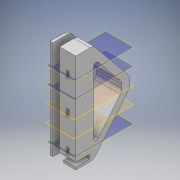
# Autodesk Inventor part: bumper_backright
Saved by Autodesk Inventor 2018 (Build 220112000, 112)
## iProperties
Created: 2019-04-08
Part Number: bumper_backright
Material: Generic
Document SubType Name: Modeling
Designer: bitbots
Density: 1 g/cm^3
Appearance: Default
Author: bitbots
Autodesk Inventor part; units mm, degrees
ref_plane "YZ Plane" through (0, 0, 0) normal (1, 0, 0) x (0, 1, 0)
ref_plane "XZ Plane" through (0, 0, 0) normal (0, 1, 0) x (-1, 0, 0)
ref_plane "XY Plane" through (0, 0, 0) normal (0, 0, 1) x (1, 0, 0)
sketch "Sketch1" plane through (0, 0, 0) normal (0, 1, 0) x (-1, 0, 0)
  line L0 (0, 0) -> (-19, 0)
  line L1 (-19, 0) -> (-19, -73)
  line L2 (-19, -73) -> (0, -73)
  line L3 (0, -73) -> (0, 0)
  dimension "d0" = 19
  dimension "d1" = 73
  constraints: 8 end point, 2 parallel, 1 horizontal, 1 perpendicular
  measures "d0" distance of L2.end L1.end
  measures "d1" distance of L1.end L0.end
extrude "Extrusion1" add sketch "Sketch1" along normal blind 13
sketch "Sketch2" plane through (19, 0, 0) normal (1, 0, 0) x (0, 0, -1)
  line L0 (0, 13) -> (0, 43) construction
  line L1 (0, 43) -> (205, 43) construction
  line L2 (0, 13) -> (0, 13.5) construction
  line L3 (0, 0) -> (0, 13) construction
  line L4 (0, 13) -> (0, 13) construction
  line L5 (0, 13) -> (73, 13) construction
  line L6 (0, 13) -> (0, 13) construction
  line L7 (0, 13) -> (73, 13) construction
  line L8 (0, 13) -> (73, 13) construction
  line L9 (36.5, 13) -> (36.5, 43) construction
  line L10 (36.5, 43) -> (0, 13) construction
  line L11 (73, 13) -> (36.5, 43) construction
  line L12 (36.5, 43) -> (30.3197, 37.9203) construction
  line L13 (30.3197, 37.9203) -> (33.4945, 34.0576) construction
  line L14 (33.4945, 34.0576) -> (7.8744, 13) construction
  line L15 (36.5, 43) -> (42.6803, 37.9203) construction
  line L16 (42.6803, 37.9203) -> (39.5055, 34.0576) construction
  line L17 (33.4945, 34.0576) -> (39.5055, 34.0576)
  line L18 (36.5, 43) -> (0, 13)
  line L19 (0, 13) -> (7.8744, 13)
  line L20 (7.8744, 13) -> (33.4945, 34.0576)
  line L21 (73, 13) -> (0, 13) construction
  line L22 (73, 13) -> (0, 13) construction
  line L23 (73, 13) -> (0, 13) construction
  line L24 (36.5, 43) -> (73, 13) construction
  line L25 (39.5055, 34.0576) -> (65.1256, 13) construction
  line L26 (36.5, 43) -> (73, 13)
  line L27 (73, 13) -> (65.1256, 13)
  line L28 (65.1256, 13) -> (39.5055, 34.0576)
  dimension "d4" = 30
  dimension "d5" = 205
  dimension "d6" = 0.5
  dimension "d7" = 0
  dimension "d8" = 0
  dimension "d9" = 73
  dimension "d10" = 0
  dimension "d11" = 8
  dimension "d12" = 5
  dimension "d13" = 8
  dimension "d14" = 5
  constraints: 54 end point, 6 collinear, 6 point on line, 6 symmetric about line, 4 perpendicular, 3 horizontal, 1 midpoint, 1 vertical
  measures "d4" distance of L0.start L0.end
  measures "d5" distance of L0.end L1.end
  measures "d6" distance of L0.start L2.end
  measures "d7" distance of L0.start L4.end
  measures "d8" distance between parallel lines of L4 L6
  measures "d9" distance of L6.end L7.end
  measures "d10" distance between parallel lines of L7 L8
  measures "d11" distance of L9.end L12.end
  measures "d12" distance of L12.end L13.end
  measures "d13" distance of L9.end L15.end
  measures "d14" distance of L15.end L16.end
extrude "Extrusion2" add sketch "Sketch2" against normal up to surface (19 mm away)
fillet "Fillet1" radius 10 1 edges at (9.5, 43, -36.5)
fillet "Fillet4" radius 2 2 edges at (9.5, 13, -7.8744) (9.5, 13, -65.1256)
fillet "Fillet5" radius 5 2 edges at (9.5, 13, -73) (9.5, 13, 0)
sketch "Sketch3" plane through (0, 0, 0) normal (0, -1, 0) x (1, 0, 0)
  line L0 (0, -73) -> (0, 0) construction
  line L1 (0, -73) -> (2, -73) construction
  line L2 (19, -73) -> (0, -73) construction
  line L3 (2, -73) -> (2, 0)
  line L4 (0, 0) -> (19, 0) projected
  line L5 (2, -73) -> (7, -73) construction
  line L6 (7, -73) -> (7, 0)
  line L7 (7, -73) -> (80, -73) construction
  line L8 (7, -73) -> (2, -73)
  line L9 (7, 0) -> (2, 0)
  dimension "d24" = 2
  dimension "d25" = 5
  dimension "d26" = 90
  constraints: 14 end point, 4 point on line, 2 collinear, 1 horizontal, 1 perpendicular, 1 vertical
  measures "d24" distance of L0.start L1.end
  measures "d25" distance of L1.end L5.end
  measures "d26" angle of L7 L6
extrude "Extrusion3" cut sketch "Sketch3" against normal blind 10
sketch "Sketch5" plane through (0, 10, 0) normal (0, -1, 0) x (1, 0, 0)
  line L0 (7, 0) -> (7, -73) projected
  line L1 (2, -73) -> (2, 0) projected
  line L2 (7, 0) -> (2, 0)
  line L3 (2, 0) -> (2, -18)
  line L4 (2, -18) -> (7, -18)
  line L5 (7, -18) -> (7, 0)
  point P0 (0, 0)
  dimension "d31" = 18
  constraints: 8 end point, 2 parallel, 1 horizontal, 1 perpendicular, 1 point on line
  measures "d31" distance of L3.end L2.end
extrude "Extrusion5" cut sketch "Sketch5" against normal up to next
sketch "Sketch6" plane through (0, 0, -73) normal (-1, 0, 0) x (0, 0, 1)
  circle A0 centre (9.0852, 5) radius 1.4
  circle A1 centre (33.5852, 5) radius 1.4
  circle A2 centre (58.0852, 5) radius 1.4
  point P0 (73, 0)
  constraints: 3 centre point, 6 other
extrude "Extrusion6" cut sketch "Sketch6" against normal blind 11.995
sketch "Sketch9" plane through (11.995, 5, -14.9148) normal (-1, 0, 0) x (0, 0, 1)
  circle A0 centre (0, 0) radius 3.002 construction
  circle A1 centre (0, 0) radius 1.4 construction
  line L0 (0, 0) -> (0, 3.002) construction
  line L1 (0, 3.002) -> (2.5998, 1.501)
  line L2 (2.5998, 1.501) -> (2.5998, -1.501)
  line L3 (2.5998, -1.501) -> (0, -3.002)
  line L4 (0, -3.002) -> (-2.5998, -1.501)
  line L5 (-2.5998, -1.501) -> (-2.5998, 1.501)
  line L6 (-2.5998, 1.501) -> (0, 3.002)
  line L7 (-58.0852, -5) -> (14.9148, -5) projected
  line L8 (-2.5998, -1.501) -> (-2.5998, -5)
  line L9 (14.9148, -5) -> (-58.0852, -5) projected
  line L10 (2.5998, -1.501) -> (2.5998, -5)
  line L11 (2.5998, -1.501) -> (6.0988, -1.501) construction
  line L12 (2.5998, -5) -> (-2.5998, -5)
  dimension "d38" = 6.004
  dimension "d41" = 90
  constraints: 22 end point, 2 perpendicular, 2 point on line, 1 coincident, 1 collinear, 1 horizontal, 1 vertical, 1 vertical alignment, 15 other
  measures "d41" angle of L10 L11
extrude "Extrusion7" cut sketch "Sketch9" against normal blind 2.005
sketch "Sketch10" plane through (14, 5, -14.9148) normal (-1, 0, 0) x (0, 0, 1)
  circle A0 centre (0, 0) radius 1.4 projected
  line L0 (2.5998, -5) -> (-2.5998, -5) projected
  line L1 (2.5998, 1.501) -> (2.5998, -5) projected
  line L2 (0, 3.002) -> (2.5998, 1.501) projected
  line L3 (-2.5998, 1.501) -> (0, 3.002) projected
  line L4 (-2.5998, -5) -> (-2.5998, 1.501) projected
  point P0 (14.9148, -5)
extrude "Extrusion8" cut sketch "Sketch10" against normal blind 2 contours A0
ref_plane "Work Plane3" through (0, 5, -14.9148) normal (0, 0, -1) x (1, 0, 0)
ref_plane "Work Plane4" through (0, 5, -39.4148) normal (0, 0, 1) x (1, 0, 0)
ref_plane "Work Plane5" through (0, 5, -63.9148) normal (0, 0, -1) x (1, 0, 0)
ref_plane "Work Plane6" through (0, 5, -27.1648) normal (0, 0, -1) x (1, 0, 0)
ref_plane "Work Plane7" through (0, 5, -51.6648) normal (0, 0, 1) x (1, 0, 0)
mirror "Mirror3" about plane through (0, 5, -27.1648) normal (0, 0, -1) of "Extrusion8", "Extrusion7"
mirror "Mirror4" about plane through (0, 5, -51.6648) normal (0, 0, 1) of "Mirror3"
fillet "Fillet6" radius 5 2 edges at (9.5, 34.0576, -39.5055) (9.5, 34.0576, -33.4945)
sketch "Sketch11" plane through (0, 0, 0) normal (0, -1, 0) x (1, 0, 0)
  line L0 (7, -73) -> (2, -73) construction
  line L1 (7, -73) -> (7, -71) construction
  line L2 (7, -73) -> (9, -73) construction
  line L3 (19, -42.8497) -> (19, -71.1748) projected
  line L4 (7, -71) -> (19, -71)
  line L5 (19, -71) -> (19, -68)
  line L6 (19, -68) -> (7, -68)
  line L7 (7, -68) -> (7, -71)
  point P0 (0, 0)
  dimension "d48" = 2
  dimension "d49" = 90
  dimension "d50" = 3
  constraints: 12 end point, 2 horizontal, 2 parallel, 2 perpendicular, 1 point on line, 1 vertical
  measures "d48" distance of L0.start L1.end
  measures "d49" angle of L2 L1
  measures "d50" distance of L5.end L4.end
extrude "Extrusion9" cut sketch "Sketch11" against normal blind 10
sketch "Sketch12" plane through (19, 10.6374, -73) normal (0, 0, -1) x (-1, 0, 0)
  line L0 (12, -10.6374) -> (0, -10.6374) projected
  line L1 (0, -0.6374) -> (12, -0.6374) projected
  line L2 (12, -10.6374) -> (9, -10.6374)
  line L3 (9, -10.6374) -> (9, -0.6374)
  line L4 (9, -0.6374) -> (12, -0.6374)
  line L5 (12, -0.6374) -> (12, -10.6374)
  point P0 (19, -10.6374)
  dimension "d53" = 3
  constraints: 8 end point, 2 parallel, 1 horizontal, 1 perpendicular, 1 point on line
  measures "d53" distance of L3.end L4.end
extrude "Extrusion10" cut sketch "Sketch12" against normal up to next
body "Solid1"
